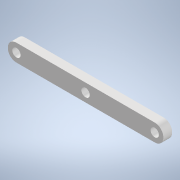
# Autodesk Inventor part: s_arm
Saved by Autodesk Inventor 2020 (Build 240168000, 168)
## iProperties
Created: 2019-10-17
Part Number: s_arm
Material: Generic
Document SubType Name: Modeling
Designer: jesse
Density: 1 g/cm^3
Appearance: Default
Author: jesse
Autodesk Inventor part; units mm, degrees
ref_plane "YZ Plane" through (0, 0, 0) normal (1, 0, 0) x (0, 1, 0)
ref_plane "XZ Plane" through (0, 0, 0) normal (0, 1, 0) x (-1, 0, 0)
ref_plane "XY Plane" through (0, 0, 0) normal (0, 0, 1) x (1, 0, 0)
sketch "Sketch1" plane through (0, 0, 0) normal (0, 0, 1) x (1, 0, 0)
  line L0 (0, 0) -> (55.7735, 0)
  line L1 (55.7735, 0) -> (55.7735, 6.175)
  line L2 (55.7735, 6.175) -> (0, 6.175)
  line L3 (0, 6.175) -> (0, 0)
  line L4 (27.8868, 6.175) -> (27.8868, 0) construction
  circle A0 centre (27.8868, 3.0875) radius 1.5
  line L5 (3.0875, 6.175) -> (3.0875, 0) construction
  line L6 (52.686, 6.175) -> (52.686, 0) construction
  circle A1 centre (3.0875, 3.0875) radius 1.5
  circle A2 centre (52.686, 3.0875) radius 1.5
  line L7 (3.0875, 3.0875) -> (0, 3.0875) construction
  line L8 (52.686, 3.0875) -> (55.7735, 3.0875) construction
  line L9 (54.1985, 3.0875) -> (54.1985, 0) construction
  dimension "d4" = 3
  dimension "d8" = 49.5986
  dimension "d10" = 6.175
  constraints: 20 end point, 7 midpoint, 6 point on line, 4 perpendicular, 3 centre point, 2 equal length, 2 equal radius, 2 parallel, 1 horizontal
  measures "d4" diameter of A2
  measures "d8" distance between parallel lines of L5 L6
  measures "d10" distance between parallel lines of L0 L2
extrude "Extrusion1" add sketch "Sketch1" along normal blind 3.175
fillet "Fillet1" radius 3 4 edges at (0, 6.175, 1.5875) (0, 0, 1.5875) (55.7735, 6.175, 1.5875) (55.7735, 0, 1.5875)
equation "\"d4\" = hole_size"
equation "\"d5\" = hole_size"
equation "\"arm_length\" = support_length"
equation "\"hole_size\" = 3"
equation "\"support_length\" = 58.42"
body "Solid1"
